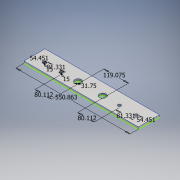
# Autodesk Inventor part: 1021sidenomotor
Saved by Autodesk Inventor 2017 (Build 210142000, 142)
## iProperties
Created: 2016-10-21
Part Number: 1021sidenomotor
Material: Aluminum 6061
Document SubType Name: Sheet Metal
Designer: aesen
Density: 2.7 g/cm^3
Sheet Metal Rule: Default_mm
Appearance: Aluminum - Flat
Author: aesen
Autodesk Inventor part; units mm, degrees
ref_plane "YZ Plane" through (0, 0, 0) normal (1, 0, 0) x (0, 1, 0)
ref_plane "XZ Plane" through (0, 0, 0) normal (0, 1, 0) x (-1, 0, 0)
ref_plane "XY Plane" through (0, 0, 0) normal (0, 0, 1) x (1, 0, 0)
sketch "Sketch1" plane through (0, 0, 0) normal (0, 0, 1) x (1, 0, 0)
  line L0 (-275.8826, -44.4336) -> (-275.8826, 56.8164)
  circle A0 centre (-221.4315, 0.0164) radius 7.5
  circle A1 centre (-140.1005, 0.0164) radius 7.5
  circle A2 centre (-59.9889, 0.0164) radius 15.875
  line L1 (-275.8826, 56.8164) -> (-0.4732, 56.8164)
  line L2 (-275.8826, -44.4336) -> (-0.4514, -44.4336)
  line L3 (274.9799, -44.4336) -> (-0.4514, -44.4336)
  line L4 (274.9799, 56.8164) -> (-0.4732, 56.8164)
  line L5 (274.9799, -44.4336) -> (274.9799, 56.8164)
  circle A3 centre (220.5289, 0.0164) radius 7.5
  circle A4 centre (139.1979, 0.0164) radius 7.5
  circle A5 centre (59.0863, 0.0164) radius 15.875
  point P0 (0, 0)
  dimension "d0" = 15
  dimension "d1" = 15
  dimension "d2" = 31.75
  dimension "d8" = 550.8625
  dimension "d14" = 80.1116
  dimension "d16" = 119.0752
  dimension "d17" = 80.1116
  dimension "d23" = 81.331
  dimension "d24" = 81.331
  dimension "d27" = 54.451
  dimension "d28" = 54.4511
  constraints: 12 end point, 6 centre point, 1 horizontal
  measures "d0" diameter of A0
  measures "d1" diameter of A1
  measures "d2" diameter of A2
  measures "d8" distance between parallel lines of L0 L5
  measures "d14" distance of A2.centre A1.centre
  measures "d16" distance of A5.centre A2.centre
  measures "d17" distance of A4.centre A5.centre
  measures "d23" distance of A3.centre A4.centre
  measures "d24" distance of A1.centre A0.centre
  measures "d27" distance from line of L5 A3.centre
  measures "d28" distance from line of L0 A0.centre
extrude "Extrusion1" add sketch "Sketch1" along normal blind 9.525
equation "\"BendRadius\" = Thickness"
equation "\"BendReliefWidth\" = Thickness"
equation "\"BendReliefDepth\" = 0.5 * Thickness"
equation "\"CornerReliefSize\" = 4 * Thickness"
equation "\"MinimumRemnant\" = 2 * Thickness"
equation "\"TransitionRadius\" = BendRadius"
equation "\"JacobiRadiusSize\" = BendRadius"
equation "\"GapSize\" = Thickness"
equation "\"Thickness\" = 0.5"
body "Solid1"
